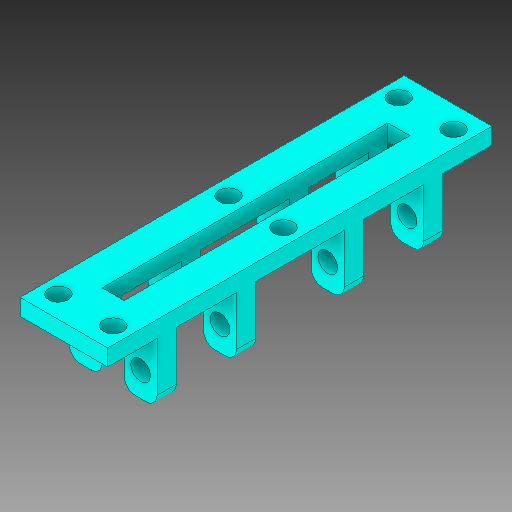
# Autodesk Inventor part: a臂鎖
Saved by Autodesk Inventor 2019 (Build 230136000, 136)
## iProperties
Created: 2020-03-15
Part Number: a臂鎖
Material: 一般
Document SubType Name: Modeling
Designer: 吳昇峻
Density: 1 g/cm^3
Appearance: 預設
Author: 吳昇峻
Autodesk Inventor part; units mm, degrees
ref_plane "YZ Plane" through (0, 0, 0) normal (1, 0, 0) x (0, 1, 0)
ref_plane "XZ Plane" through (0, 0, 0) normal (0, 1, 0) x (-1, 0, 0)
sketch "草圖1" plane through (0, 0, 0) normal (0, 1, 0) x (-1, 0, 0)
  line L0 (403.4401, 81.3797) -> (399.9401, 81.3797) construction
  line L1 (399.9401, 81.3797) -> (399.9401, 70.3797) construction
  line L2 (399.9401, 70.3797) -> (403.4401, 70.3797) construction
  line L3 (403.4401, 70.3797) -> (403.4401, 81.3797) construction
  line L4 (403.4401, 81.3797) -> (399.9401, 70.3797) construction
  line L5 (399.9401, 81.3797) -> (403.4401, 70.3797) construction
  line L6 (403.4401, 70.3797) -> (404.6901, 70.3797)
  line L7 (398.6901, 70.3797) -> (403.4401, 70.3797)
  line L8 (403.4401, 81.3797) -> (404.6901, 81.3797)
  line L9 (404.6901, 84.8797) -> (398.6901, 84.8797)
  line L10 (398.6901, 81.3797) -> (403.4401, 81.3797)
  line L11 (404.6901, 93.8797) -> (398.6901, 93.8797)
  line L12 (398.6901, 93.8797) -> (398.6901, 57.8797)
  line L13 (404.6901, 57.8797) -> (404.6901, 93.8797)
  line L14 (404.6901, 93.8797) -> (398.6901, 57.8797) construction
  line L15 (398.6901, 93.8797) -> (404.6901, 57.8797) construction
  line L16 (401.6901, 84.8797) -> (401.6901, 89.8797) construction
  circle A0 centre (401.6901, 89.8797) radius 1.8
  line L17 (401.6901, 75.8797) -> (401.6901, 41.6777) construction
  circle A1 centre (401.6901, 58.7787) radius 1.8
  line L18 (404.6901, 66.8797) -> (398.6901, 66.8797)
  line L19 (403.4401, 36.1777) -> (399.9401, 36.1777) construction
  line L20 (399.9401, 36.1777) -> (399.9401, 47.1777) construction
  line L21 (399.9401, 47.1777) -> (403.4401, 47.1777) construction
  line L22 (403.4401, 47.1777) -> (403.4401, 36.1777) construction
  line L23 (403.4401, 36.1777) -> (399.9401, 47.1777) construction
  line L24 (399.9401, 36.1777) -> (403.4401, 47.1777) construction
  line L25 (403.4401, 47.1777) -> (404.6901, 47.1777)
  line L26 (398.6901, 47.1777) -> (403.4401, 47.1777)
  line L27 (403.4401, 36.1777) -> (404.6901, 36.1777)
  line L28 (404.6901, 32.6777) -> (398.6901, 32.6777)
  line L29 (398.6901, 36.1777) -> (403.4401, 36.1777)
  line L30 (404.6901, 23.6777) -> (398.6901, 23.6777)
  line L31 (398.6901, 23.6777) -> (398.6901, 59.6777)
  line L32 (404.6901, 59.6777) -> (404.6901, 23.6777)
  line L33 (404.6901, 23.6777) -> (398.6901, 59.6777) construction
  line L34 (398.6901, 23.6777) -> (404.6901, 59.6777) construction
  line L35 (401.6901, 32.6777) -> (401.6901, 27.6777) construction
  circle A2 centre (401.6901, 27.6777) radius 1.8
  circle A3 centre (401.6901, 58.7787) radius 1.8
  line L36 (404.6901, 50.6777) -> (398.6901, 50.6777)
  line L37 (404.6901, 66.8797) -> (398.6901, 66.8797)
  line L38 (398.6901, 66.8797) -> (398.6901, 50.6777)
  line L39 (398.6901, 50.6777) -> (404.6901, 50.6777)
  line L40 (404.6901, 50.6777) -> (404.6901, 66.8797)
  line L41 (401.6901, 58.7787) -> (391.6591, 58.7787) construction
  line L42 (396.6746, 58.7787) -> (396.6746, 63.5433) construction
  line L43 (391.6591, 58.7787) -> (401.6901, 58.7787) construction
  line L44 (398.6901, 66.8797) -> (394.6591, 66.8797)
  line L45 (398.6901, 50.6777) -> (394.6591, 50.6777)
  point P0 (0, 0)
  point P1 (398.1901, 70.3797)
  point P2 (398.1901, 81.3797)
  point P3 (398.1901, 47.1777)
  point P4 (398.1901, 36.1777)
  dimension "d8" = 11
  dimension "d34" = 36
  dimension "d35" = 5
  dimension "d37" = 3.6
  dimension "d49" = 34.202
  dimension "d50" = 3.6
  dimension "d61" = 10.031
  constraints: 92 end point, 20 point on line, 8 horizontal, 8 midpoint, 5 parallel, 4 centre point, 4 symmetric about line, 3 perpendicular, 3 vertical, 2 coincident, 1 collinear
  measures "d8" distance of L1.end L0.end
  measures "d34" distance of L12.end L11.end
  measures "d35" distance of L16.start L16.end
  measures "d37" diameter of A0
  measures "d49" distance of L17.start L17.end
  measures "d50" diameter of A1
  measures "d61" distance of L41.start L41.end
extrude "擠出8" add sketch "草圖1" along normal blind 3
extrude "擠出9" add sketch "草圖1" against normal blind 11 contours L6 L13 L18 L12 L7 | L8 L10 L12 L9 L13 | L32 L25 L26 L31 L36 | L32 L28 L31 L29 L27
fillet "圓角4" radius 2 8 edges at (-404.6901, -11, 34.4277) (-398.6901, -11, 34.4277) (-404.6901, -11, 48.9277) (-398.6901, -11, 48.9277) (-404.6901, -11, 68.6297) (-398.6901, -11, 68.6297) (-398.6901, -11, 83.1297) (-404.6901, -11, 83.1297)
sketch "草圖4" plane through (-398.6901, 0, 32.6777) normal (0, 0, -1) x (-1, 0, 0)
  line L0 (0, 0) -> (6, 0) construction
  line L1 (6, 0) -> (3, 0) construction
  line L2 (3, 0) -> (3, -6.5) construction
  circle A0 centre (3, -6.5) radius 1.8
  point P0 (-398.6901, 0)
  dimension "d57" = 6.5
  dimension "d58" = 3.6
  constraints: 4 end point, 1 centre point, 1 coincident, 1 midpoint, 1 perpendicular
  measures "d57" distance of L1.end L2.end
  measures "d58" diameter of A0
extrude "擠出10" cut sketch "草圖4" against normal through all
ref_plane "工作平面4" through (-396.6746, 0, 58.7787) normal (1, 0, 0) x (0, 0, -1)
mirror "鏡射2" about plane through (-396.6746, 0, 58.7787) normal (1, 0, 0) of "擠出8", "擠出9", "擠出10", "圓角4"
sketch "草圖8" plane through (0, 0, 0) normal (0, 1, 0) x (-1, 0, 0)
  line L0 (398.6901, 32.6777) -> (398.6901, 23.6777) projected
  line L1 (394.6591, 32.6777) -> (394.6591, 23.6777) projected
  line L2 (398.6901, 93.8797) -> (398.6901, 84.8797) projected
  line L3 (394.6591, 93.8797) -> (394.6591, 84.8797) projected
  line L4 (404.6901, 93.8797) -> (398.6901, 93.8797) projected
  line L5 (388.6591, 93.8797) -> (394.6591, 93.8797) projected
  line L6 (398.6901, 93.8797) -> (394.6591, 93.8797)
  line L7 (398.6901, 84.8797) -> (394.6591, 84.8797)
  line L8 (398.6901, 32.6777) -> (394.6591, 32.6777)
  line L9 (398.6901, 23.6777) -> (394.6591, 23.6777)
  point P0 (0, 0)
  constraints: 8 end point, 4 horizontal
extrude "擠出13" add sketch "草圖8" along normal blind 3
